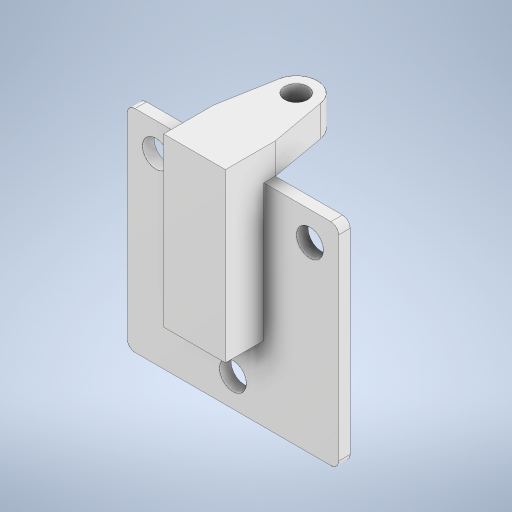
# Autodesk Inventor part: Electromagnet Gantry Plate
Saved by Autodesk Inventor 2023.2 (Build 272271030, 271C)
## iProperties
Created: 2023-04-10
Part Number: Electromagnet Gantry Plate
Material: PC/ABS Plastic
Document SubType Name: Modeling
Designer: ethan
Density: 0.357273 g/cm^3
Appearance: Smooth - White
Author: ethan
Autodesk Inventor part; units mm, degrees
ref_plane "YZ Plane" through (0, 0, 0) normal (1, 0, 0) x (0, 1, 0)
ref_plane "XZ Plane" through (0, 0, 0) normal (0, 1, 0) x (-1, 0, 0)
ref_plane "XY Plane" through (0, 0, 0) normal (0, 0, 1) x (1, 0, 0)
sketch "Sketch1" plane through (0, 0, 0) normal (0, 1, 0) x (-1, 0, 0)
  line L0 (0, 0) -> (55, 0)
  line L1 (55, 0) -> (55, -55)
  line L2 (55, -55) -> (0, -55)
  line L3 (0, -55) -> (0, 0)
  line L4 (47.55, -7.45) -> (7.45, -7.45) construction
  line L5 (7.45, -7.45) -> (7.45, -47.55) construction
  line L6 (7.45, -47.55) -> (47.55, -47.55) construction
  line L7 (47.55, -47.55) -> (47.55, -7.45) construction
  circle A0 centre (47.55, -7.45) radius 3.5
  circle A1 centre (47.55, -47.55) radius 3.5
  circle A2 centre (7.45, -47.55) radius 3.5
  circle A3 centre (7.45, -7.45) radius 3.5
  circle A4 centre (47.55, -7.45) radius 12.5 construction
  circle A5 centre (27.5, -7.45) radius 3.5
  dimension "d0" = 55
  dimension "d1" = 55
  dimension "d2" = 40.1
  dimension "d3" = 40.1
  dimension "d4" = 7
  dimension "d5" = 7
  dimension "d6" = 7
  dimension "d7" = 7
  dimension "d8" = 7.45
  dimension "d9" = 7.45
  dimension "d13" = 25
  dimension "d14" = 7
  constraints: 16 end point, 6 centre point, 5 coincident, 4 parallel, 2 horizontal, 2 perpendicular, 1 midpoint
  measures "d0" distance of L1.end L2.end
  measures "d1" distance of L0.end L1.end
  measures "d2" distance of L6.end L5.end
  measures "d3" distance of L5.end L4.end
  measures "d4" diameter of A0
  measures "d5" diameter of A3
  measures "d6" diameter of A1
  measures "d7" diameter of A2
  measures "d8" distance between parallel lines of L1 L7
  measures "d9" distance from line of L2 L5.end
  measures "d13" diameter of A4
  measures "d14" diameter of A5
extrude "Extrusion1" add sketch "Sketch1" along normal blind 3 contours L0 L1 L2 L3 | A0 | A3
fillet "Fillet1" radius 2 4 edges at (-55, 1.5, 0) (0, 1.5, 0) (-55, 1.5, -55) (0, 1.5, -55)
sketch "Sketch3" plane through (0, 0, -53) normal (1, 0, 0) x (0, 0, -1)
  line L0 (-13, 0) -> (-13, -20) construction
  line L1 (12, -20) -> (-13, -20) construction
  line L2 (-13, 0) -> (-33, 0) construction
  line L3 (-33, 0) -> (-33, -20) construction
  line L4 (-33, -20) -> (-13, -20) construction
  line L5 (-13, -20) -> (-13, 0) construction
  line L6 (2, 0) -> (-13, 0) construction
  line L7 (-13, 0) -> (-33, -20) construction
  line L8 (-33, -10) -> (-13, -10) projected
  circle A0 centre (-23, -10) radius 5
  point P0 (-53, 0)
  point P1 (2, -20)
  dimension "d25" = 10
  constraints: 10 end point, 2 parallel, 1 centre point, 1 horizontal, 1 midpoint, 1 perpendicular
  measures "d25" diameter of A0
extrude "Extrusion3" cut sketch "Sketch3" against normal blind 12
sketch "Sketch4" plane through (-55, 0, -2) normal (-1, 0, 0) x (0, 0, 1)
  circle A0 centre (-28, -10) radius 5 projected
  circle A1 centre (-28, -10) radius 2.75
  point P0 (2, 0)
  dimension "d30" = 5.5
  constraints: 1 centre point, 1 coincident
  measures "d30" diameter of A1
extrude "Extrusion4" cut sketch "Sketch4" against normal blind 12 contours A0 | A1
extrude "Extrusion5" cut sketch "Sketch4" against normal through all contours A1
sketch "Sketch5" plane through (-53, 3, 0) normal (0, 0, 1) x (1, 0, 0)
  line L0 (35.5, -3) -> (35.5, -23) construction
  line L1 (15.5, -3) -> (15.5, -23) construction
  line L2 (35.5, -3) -> (15.5, -3) construction
  line L3 (15.5, -3) -> (15.5, -23) construction
  line L4 (15.5, -23) -> (35.5, -23) construction
  line L5 (35.5, -23) -> (35.5, -3) construction
  line L6 (15.5, -23) -> (35.5, -23) construction
  line L7 (15.5, -3) -> (-2, -3) construction
  line L8 (35.5, -23) -> (15.5, -3) construction
  circle A0 centre (25.5, -13) radius 5
  circle A1 centre (25.5, -13) radius 2.75
  point P0 (53, -3)
  dimension "d33" = 10
  dimension "d34" = 5.5
  constraints: 10 end point, 2 centre point, 2 parallel, 1 coincident, 1 horizontal, 1 midpoint, 1 perpendicular
  measures "d33" diameter of A0
  measures "d34" diameter of A1
extrude "Extrusion6" cut sketch "Sketch5" against normal blind 12 contours A0 | A1
sketch "Sketch6" plane through (0, 0, 0) normal (0, -1, 0) x (1, 0, 0)
  circle A0 centre (-7.45, -47.55) radius 3.5 projected
  circle A1 centre (-47.55, -47.55) radius 3.5 projected
  circle A2 centre (-27.5, -7.45) radius 3.5 projected
  line L0 (-35.55, -63) -> (-35.55, -19.45)
  line L1 (-35.55, -19.45) -> (-19.45, -19.45)
  line L2 (-19.45, -19.45) -> (-19.45, -63)
  line L3 (-2, -55) -> (-53, -55) projected
  line L4 (-19.45, -63) -> (-35.55, -63)
  point P0 (0, 0)
  constraints: 8 end point, 1 parallel, 1 perpendicular
extrude "Extrusion8" add sketch "Sketch6" along normal blind 10 contours L0 L3 L2 L4 | L0 L1 L2 L3
sketch "Sketch7" plane through (0, 0, 0) normal (0, 1, 0) x (1, 0, 0)
  line L0 (-19.45, 63) -> (-19.45, 53.4092)
  line L1 (-35.55, 19.45) -> (-35.55, 63) projected
  line L2 (-19.45, 55) -> (-35.55, 55)
  line L3 (-35.55, 55) -> (-35.55, 63)
  line L4 (-35.55, 63) -> (-19.45, 63)
  line L5 (-19.45, 63) -> (-19.45, 55)
  point P0 (0, 0)
  point P1 (-53, 55)
  constraints: 10 end point, 2 parallel, 1 horizontal, 1 perpendicular, 1 point on line
extrude "Extrusion9" add sketch "Sketch7" along normal blind 22
sketch "Sketch8" plane through (-19.45, -10, -63) normal (0, 0, -1) x (-1, 0, 0)
  line L0 (-19.45, 13) -> (27.4883, 13)
  line L1 (33.55, 13) -> (-17.45, 13) projected
  line L2 (8.05, 13) -> (8.05, 26.475) construction
  circle A0 centre (8.05, 26.475) radius 5.525
  line L3 (0, 32) -> (16.1, 32) projected
  line L4 (0, 13) -> (2.6131, 27.4577)
  line L5 (16.1, 13) -> (13.4869, 27.4577)
  line L6 (0, 10) -> (0, 13) projected
  line L7 (0, 13) -> (0, 32)
  line L8 (16.1, 32) -> (0, 32) projected
  line L9 (0, 32) -> (16.1, 32)
  line L10 (16.1, 32) -> (16.1, 13)
  point P0 (-19.45, 10)
  point P1 (8.05, 32)
  point P2 (2.6131, 27.4577)
  dimension "d50" = 13.475
  constraints: 14 end point, 3 point on line, 3 tangent, 2 collinear, 1 centre point, 1 coincident, 1 midpoint, 1 perpendicular, 1 vertical
  measures "d50" distance of L2.start L2.end
extrude "Extrusion10" cut sketch "Sketch8" against normal through all contours L7 L3 A0 L4 | L5 A0 L3 L10
sketch "Sketch9" plane through (-19.45, -10, -63) normal (0, 0, -1) x (-1, 0, 0)
  line L0 (0, 0) -> (0, 13) projected
  line L1 (16.1, 13) -> (16.1, 10) projected
  line L2 (0, 13) -> (16.1, 13)
  line L3 (4.55, 13) -> (11.55, 13) projected
  line L4 (8.05, 13) -> (8.05, 26.475)
  circle A0 centre (8.05, 26.475) radius 3
  point P0 (-19.45, 10)
  dimension "d54" = 13.475
  dimension "d55" = 6
  constraints: 4 end point, 1 centre point, 1 coincident, 1 midpoint, 1 perpendicular, 1 vertical
  measures "d54" distance of L4.start L4.end
  measures "d55" diameter of A0
extrude "Extrusion11" cut sketch "Sketch9" against normal through all
equation "\"d1\" = d0"
equation "\"d3\" = d2"
equation "\"d5\" = d4"
equation "\"d6\" = d4"
equation "\"d7\" = d4"
equation "\"d8\" = -0.5 * d2 + 0.5 * d0"
equation "\"d9\" = -0.5 * d3 + 0.5 * d1"
equation "\"d14\" = d4"
body "Solid1"
